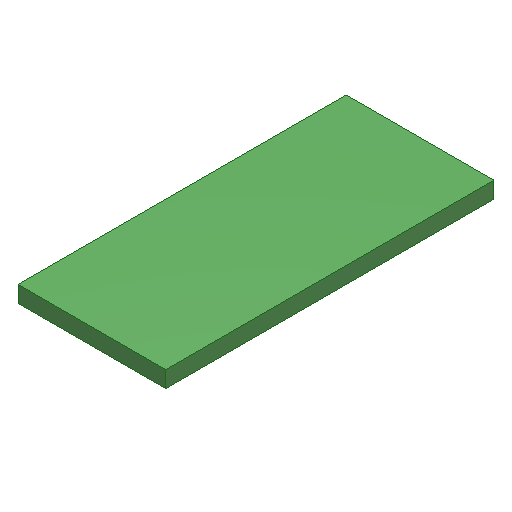
# Autodesk Inventor part: ASSEMBLY_PCB_Line_sensor
Saved by Autodesk Inventor 2026.1 (Build 301233000, 233)
## iProperties
Created: 2016-04-16
Part Number: ASSEMBLY_PCB_Line_sensor
Material: Ogólny
Document SubType Name: Modeling
Designer: Andrzej
Density: 1 g/cm^3
Appearance: Gładki - ciemna zieleń leśna
Mass: 0.19377 g
Surface Area: 4.363 cm^2
Volume: 0.19377 cm^3
Author: Andrzej
Autodesk Inventor part; units mm, degrees
ref_plane "YZ Plane" through (0, 0, 0) normal (1, 0, 0) x (0, 1, 0)
ref_plane "XZ Plane" through (0, 0, 0) normal (0, 1, 0) x (-1, 0, 0)
ref_plane "XY Plane" through (0, 0, 0) normal (0, 0, 1) x (1, 0, 0)
sketch "Szkic1" plane through (0, 0, 0) normal (0, 0, 1) x (1, 0, 0)
  line L0 (-3.9202, 0.9902) -> (-1.2202, 0.9902)
  line L1 (-1.2202, 0.9902) -> (-1.2202, -2.4098)
  line L2 (-1.2202, -2.4098) -> (-3.9202, -2.4098)
  line L3 (-3.9202, -2.4098) -> (-3.9202, 0.9902)
  point P0 (0, 0)
  dimension "d0" = 2.7
  dimension "d1" = 3.4
  constraints: 8 end point, 2 parallel, 1 horizontal, 1 perpendicular
  measures "d0" distance of L1.end L2.end
  measures "d1" distance of L0.end L1.end
extrude "Wyciągnięcie proste1" add sketch "Szkic1" along normal blind 1.5
sketch "Szkic2" plane through (0, 0, 1.5) normal (0, 0, 1) x (1, 0, 0)
  line L0 (-8.2202, 2.4902) -> (0.7798, 2.4902)
  line L1 (0.7798, 2.4902) -> (0.7798, -17.5098)
  line L2 (0.7798, -17.5098) -> (-8.2202, -17.5098)
  line L3 (-8.2202, -17.5098) -> (-8.2202, 2.4902)
  line L4 (-1.2202, 0.9902) -> (-3.9202, 0.9902) projected
  line L5 (-3.9202, 0.9902) -> (-3.9202, -2.4098) projected
  line L6 (-3.9202, -2.4098) -> (-1.2202, -2.4098) projected
  line L7 (-1.2202, -2.4098) -> (-1.2202, 0.9902) projected
  point P0 (0, 0)
  dimension "d4" = 9
  dimension "d5" = 20
  dimension "d7" = 1.5
  dimension "d10" = 2
  constraints: 8 end point, 2 parallel, 1 horizontal, 1 perpendicular
  measures "d4" distance of L1.end L2.end
  measures "d5" distance of L0.end L1.end
  measures "d7" distance between parallel lines of L0 L4
  measures "d10" distance between parallel lines of L1 L7
extrude "Wyciągnięcie proste2" add sketch "Szkic2" along normal blind 1 contours L0 L1 L2 L3 | L7 L6 L5 L4
